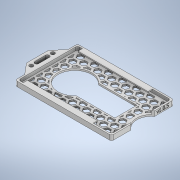
# Autodesk Inventor part: badge
Saved by Autodesk Inventor 2022 (Build 260153000, 153)
## iProperties
Created: 2019-12-22
Part Number: badge
Material: Generic
Document SubType Name: Modeling
Designer: user
Density: 1 g/cm^3
Appearance: Default
Author: user
## iProperties of the stored document _3DPrint.ipt
Created: 2019-12-23
Part Number: _3DPrint
Material: Generic
Document SubType Name: Modeling
Designer: user
Density: 1 g/cm^3
Appearance: Default
Author: user
Autodesk Inventor part; units mm, degrees
(part 1 of 2)
ref_plane "YZ Plane" through (0, 0, 0) normal (1, 0, 0) x (0, 1, 0)
ref_plane "XZ Plane" through (0, 0, 0) normal (0, 1, 0) x (-1, 0, 0)
ref_plane "XY Plane" through (0, 0, 0) normal (0, 0, 1) x (1, 0, 0)
sketch "Sketch1" plane through (0, 0, 0) normal (0, 1, 0) x (-1, 0, 0)
  line L0 (10.6639, 24.1888) -> (-74.7361, 24.1888)
  line L1 (-74.7361, -33.7112) -> (10.6639, -33.7112)
  line L2 (12.6639, 15.2886) -> (20.5717, 5.8644)
  line L3 (21.0396, 4.5789) -> (21.0396, -14.1414)
  line L4 (20.5717, -15.427) -> (12.6639, -24.8511)
  circle A0 centre (-13.8361, -4.7612) radius 17
  line L5 (-62.6217, 4.9888) -> (-62.6217, -14.5112)
  line L6 (-60.6217, -16.5112) -> (-26.1217, -16.5112)
  line L7 (-26.1217, 6.9888) -> (-60.6217, 6.9888)
  arc A1 (-62.6217, -14.5112) -> (-60.6217, -16.5112) centre (-60.6217, -14.5112) ccw
  arc A2 (-60.6217, 6.9888) -> (-62.6217, 4.9888) centre (-60.6217, 4.9888) ccw
  line L8 (-28.5861, -0.5112) -> (-55.1217, -0.5112)
  line L9 (-55.1217, -0.5112) -> (-55.1217, -9.0112)
  line L10 (-55.1217, -9.0112) -> (-28.5861, -9.0112)
  line L11 (-28.5861, -9.0112) -> (-28.5861, -0.5112)
  line L12 (-76.7361, 6.1888) -> (-76.7361, 22.1888)
  line L13 (-76.7361, -15.7112) -> (-76.7361, -31.7112)
  line L14 (9.1639, 22.6888) -> (-73.2361, 22.6888)
  line L15 (-73.2361, -32.2112) -> (9.1639, -32.2112)
  line L16 (11.1639, -30.2112) -> (11.1639, 20.6888)
  line L17 (-75.2361, 20.6888) -> (-75.2361, 4.8633)
  line L18 (-75.2361, -30.2112) -> (-75.2361, -14.3857)
  line L19 (12.6639, 22.1888) -> (12.6639, 15.2886)
  line L20 (12.6639, -24.8511) -> (12.6639, -31.7112)
  arc A3 (-76.7361, -31.7112) -> (-74.7361, -33.7112) centre (-74.7361, -31.7112) ccw
  arc A4 (-75.2361, -30.2112) -> (-73.2361, -32.2112) centre (-73.2361, -30.2112) ccw
  arc A5 (-73.2361, 22.6888) -> (-75.2361, 20.6888) centre (-73.2361, 20.6888) ccw
  arc A6 (-74.7361, 24.1888) -> (-76.7361, 22.1888) centre (-74.7361, 22.1888) ccw
  arc A7 (12.6639, 22.1888) -> (10.6639, 24.1888) centre (10.6639, 22.1888) ccw
  arc A8 (11.1639, 20.6888) -> (9.1639, 22.6888) centre (9.1639, 20.6888) ccw
  arc A9 (9.1639, -32.2112) -> (11.1639, -30.2112) centre (9.1639, -30.2112) ccw
  arc A10 (10.6639, -33.7112) -> (12.6639, -31.7112) centre (10.6639, -31.7112) ccw
  arc A11 (20.5717, -15.427) -> (21.0396, -14.1414) centre (19.0396, -14.1414) ccw
  arc A12 (21.0396, 4.5789) -> (20.5717, 5.8644) centre (19.0396, 4.5789) ccw
  arc A13 (-76.7361, -15.7112) -> (-76.7361, 6.1888) centre (-85.0764, -4.7612) ccw
  circle A14 centre (16.6641, 5.1661) radius 1.75
  circle A15 centre (16.6641, -14.7286) radius 1.75
  line L21 (12.6639, 15.2886) -> (12.6639, -24.8511)
  line L22 (18.4257, 0.4632) -> (18.4257, -9.9334)
  line L23 (14.9257, 0.4403) -> (14.9257, -10.0946)
  arc A16 (14.9257, -10.0946) -> (18.4257, -9.9334) centre (16.6641, -9.7623) ccw
  arc A17 (18.4257, 0.4632) -> (14.9257, 0.4403) centre (16.6774, 0.1997) ccw
  point P0 (0, 0)
  point P1 (12.6639, 24.1888)
  point P2 (-76.7361, -33.7112)
  point P3 (-76.7361, 24.1888)
  point P4 (12.6639, -33.7112)
  point P5 (21.0396, -14.8693)
  point P6 (-62.6217, -16.5112)
  dimension "d19" = 18
  dimension "d20" = 34
  dimension "d26" = 2
  dimension "d28" = 7.5
  dimension "d32" = 7.5
  dimension "d33" = 7.5
  dimension "d36" = 1.5
  dimension "d37" = 1.5
  dimension "d40" = 1.5
  dimension "d41" = 2
  dimension "d84" = 54.9
  dimension "d89" = 18
  dimension "d104" = 86.4
  dimension "d110" = 13.7646
  dimension "d116" = 1.5
  dimension "d122" = 3.5
  dimension "d123" = 3.5
  dimension "d124" = 3.4423
  dimension "d125" = 3.4423
  dimension "d155" = 25
  dimension "d163" = 15.7
  dimension "d164" = 15.7
  dimension "d165" = 27.45
  dimension "d166" = 27.45
  dimension "d167" = 8.5
  dimension "d171" = 26.5357
  dimension "d173" = 39.75
  dimension "d213" = 4.0002
  dimension "d214" = 4.0002
  dimension "d219" = 140
  dimension "d221" = 140
  dimension "d246" = 4.9664
  dimension "d247" = 4.9664
  dimension "d248" = 13.5
  dimension "d249" = 1.5
  dimension "d250" = 1.5
  dimension "d251" = 4.0002
  dimension "d262" = 3.5
  dimension "d263" = 2.6139
  constraints: 48 end point, 34 point on circle, 24 tangent, 18 centre point, 13 point on line, 10 equal radius, 6 vertical, 5 parallel, 3 horizontal, 3 perpendicular, 2 collinear
  measures "d19" distance of point (-76.736, 24.189) L12.start
  measures "d20" diameter of A0
  measures "d26" radius of A1
  measures "d28" distance between parallel lines of L6 L10
  measures "d32" distance between parallel lines of L8 L7
  measures "d33" distance between parallel lines of L5 L9
  measures "d36" distance between parallel lines of L0 L14
  measures "d37" distance between parallel lines of L1 L15
  measures "d40" distance between parallel lines of L13 L18
  measures "d41" radius of A3
  measures "d84" distance between parallel lines of L15 L14
  measures "d89" distance of L13.start point (-76.736, -33.711)
  measures "d104" distance between parallel lines of L17 L16
  measures "d110" radius of A13
  measures "d116" distance between parallel lines of L17 L12
  measures "d122" diameter of A15
  measures "d123" diameter of A14
  measures "d124" distance from line of L4 A15.centre
  measures "d125" distance from line of L2 A14.centre
  measures "d155" distance from line of L16 A0.centre
  measures "d163" distance between parallel lines of L15 L6
  measures "d164" distance between parallel lines of L14 L7
  measures "d165" distance from line of L15 A0.centre
  measures "d166" distance from line of L14 A0.centre
  measures "d167" distance between parallel lines of L8 L10
  measures "d171" distance between parallel lines of L9 L11
  measures "d173" distance between parallel lines of L16 L11
  measures "d213" distance from line of L21 A14.centre
  measures "d214" distance from line of L21 A15.centre
  measures "d219" angle of L19 L2
  measures "d221" angle of L20 L4
  measures "d246" distance of A17.centre A14.centre
  measures "d247" distance of A15.centre A16.centre
  measures "d249" distance between parallel lines of L16 L19
  measures "d250" distance between parallel lines of L16 L20
  measures "d251" distance from line of L21 A16.centre
  measures "d262" distance between parallel lines of L23 L22
  measures "d263" distance from line of L3 L22.end
extrude "OutsideFrame_Ex" add sketch "Sketch1" along normal blind 4.5 contours A7 L19 L21 L20 A10 L1 A3 L13 A13 L18 A4 L15 A9 L16 A8 L14 A5 L17 L12 A6 L0
extrude "CardRidge" add sketch "Sketch1" along normal blind 1.5 contours L17 A5 L14 A8 L16 A9 L15 A4 L18 A13 | A0 L10 L11 L8 | A0 L8 L9 L10 L6 A1 L5 A2 L7 picked at (-18.0028, -4.7612)
sketch "Sketch5" plane through (73.2361, 4.5, 22.6888) normal (0, 0, -1) x (-1, 0, 0)
  line L0 (-2, 0) -> (0, 0) projected
  line L1 (79.9, 0) -> (79.9, -1)
  line L2 (0, 0) -> (82.4, 0) projected
  line L3 (15, 0) -> (79.9, 0)
  line L4 (79.9, 0) -> (79.9, -1)
  line L5 (79.9, -1) -> (15, -1)
  line L6 (15, -1) -> (15, 0)
  line L7 (0, -4.5) -> (0, 0) projected
  line L8 (82.4, -4.5) -> (82.4, 0) projected
  line L9 (0, -3) -> (82.4, -3) projected
  point P0 (73.2361, -4.5)
  dimension "d65" = 15
  dimension "d66" = 2.5
  dimension "d67" = 1
  constraints: 10 end point, 2 parallel, 1 horizontal, 1 perpendicular, 1 point on line
  measures "d65" distance between parallel lines of L7 L6
  measures "d66" distance between parallel lines of L8 L1
  measures "d67" distance between parallel lines of L5 L2
extrude "LeftSlider" add sketch "Sketch5" along normal blind 4 contours L1 L5 L6 L2
sketch "Sketch6" plane through (-9.1639, 4.5, -32.2112) normal (0, 0, 1) x (1, 0, 0)
  line L0 (83.9, 0) -> (-1.5, 0) projected
  line L1 (2.5, 0) -> (67.4, 0)
  line L2 (67.4, 0) -> (67.4, -1)
  line L3 (67.4, -1) -> (2.5, -1)
  line L4 (2.5, -1) -> (2.5, 0)
  line L5 (0, -3) -> (0, 0) projected
  line L6 (82.4, -3) -> (82.4, 0) projected
  point P0 (9.1639, -4.5)
  point P1 (0, -7.4)
  point P2 (83.7968, -7.4)
  dimension "d71" = 2.5
  dimension "d72" = 15
  dimension "d73" = 1
  constraints: 8 end point, 2 parallel, 1 horizontal, 1 perpendicular, 1 point on line, 1 other
  measures "d71" distance between parallel lines of L5 L4
  measures "d73" distance between parallel lines of L3 L0
extrude "RightSlider" add sketch "Sketch6" along normal blind 4
extrude "TopHolder" add sketch "Sketch1" along normal blind 4.5 contours L2 A12 L3 A11 L4 L21
sketch "Sketch15" plane through (76.7361, 0, -15.7112) normal (1, 0, 0) x (0, 0, -1)
  line L0 (2.0176, 4.0473) -> (13.0095, 4.0473) construction
  line L1 (13.0095, 4.0473) -> (13.0095, -1.0349) construction
  line L2 (13.0095, -1.0349) -> (2.0176, -1.0349) construction
  line L3 (2.0176, -1.0349) -> (2.0176, 4.0473) construction
  line L4 (4.0924, 3.2248) -> (3.2304, 0.9376)
  line L5 (3.2304, 0.9376) -> (2.8846, 0.9376)
  line L6 (2.8846, 0.9376) -> (2.03, 3.2248)
  line L7 (2.03, 3.2248) -> (2.4474, 3.2248)
  line L8 (2.4474, 3.2248) -> (3.0723, 1.4637)
  line L9 (3.0723, 1.4637) -> (3.6923, 3.2248)
  line L10 (3.6923, 3.2248) -> (4.0924, 3.2248)
  line L11 (6.0536, 0.9376) -> (4.5667, 0.9376)
  line L12 (4.5667, 0.9376) -> (4.5667, 1.2488)
  line L13 (4.5667, 1.2488) -> (5.1199, 1.2488)
  line L14 (5.1199, 1.2488) -> (5.1199, 3.2915)
  line L15 (5.1199, 3.2915) -> (4.5667, 3.2915)
  line L16 (4.5667, 3.2915) -> (4.5667, 3.5706)
  spline S0 degree 2 poles (4.5667, 3.5706) (4.8803, 3.5706) (5.1768, 3.7485) (5.1965, 3.9955) knots 0 0 0 1 2 2 2
  line L17 (5.1965, 3.9955) -> (5.5127, 3.9955)
  line L18 (5.5127, 3.9955) -> (5.5127, 1.2488)
  line L19 (5.5127, 1.2488) -> (6.0536, 1.2488)
  line L20 (6.0536, 1.2488) -> (6.0536, 0.9376)
  line L21 (7.2689, 0.9376) -> (6.7798, 0.9376)
  line L22 (6.7798, 0.9376) -> (6.7798, 1.5205)
  line L23 (6.7798, 1.5205) -> (7.2689, 1.5205)
  line L24 (7.2689, 1.5205) -> (7.2689, 0.9376)
  spline S1 degree 2 poles (9.7809, 2.4616) (9.7809, 1.6415) (9.3041, 0.8734) (8.8077, 0.8734) knots 0 0 0 1 2 2 2
  spline S2 degree 2 poles (8.8077, 0.8734) (8.3038, 0.8734) (7.832, 1.6564) (7.832, 2.4591) knots 0 0 0 1 2 2 2
  spline S3 degree 2 poles (7.832, 2.4591) (7.832, 3.2841) (8.3087, 4.0473) (8.8077, 4.0473) knots 0 0 0 1 2 2 2
  spline S4 degree 2 poles (8.8077, 4.0473) (9.3091, 4.0473) (9.7809, 3.2569) (9.7809, 2.4616) knots 0 0 0 1 2 2 2
  spline S5 degree 2 poles (9.2572, 1.5329) (9.3165, 1.6835) (9.3659, 2.1479) (9.3659, 2.4616) knots 0 0 0 1 2 2 2
  spline S6 degree 2 poles (9.3659, 2.4616) (9.3659, 2.7753) (9.3165, 3.2372) (9.2547, 3.3928) knots 0 0 0 1 2 2 2
  spline S7 degree 2 poles (9.2547, 3.3928) (9.193, 3.5484) (8.9781, 3.7089) (8.8077, 3.7089) knots 0 0 0 1 2 2 2
  spline S8 degree 2 poles (8.8077, 3.7089) (8.6372, 3.7089) (8.4174, 3.5484) (8.3532, 3.3878) knots 0 0 0 1 2 2 2
  spline S9 degree 2 poles (8.3532, 3.3878) (8.2914, 3.2322) (8.247, 2.758) (8.247, 2.4591) knots 0 0 0 1 2 2 2
  spline S10 degree 2 poles (8.247, 2.4591) (8.247, 2.138) (8.2865, 1.7082) (8.3507, 1.5403) knots 0 0 0 1 2 2 2
  spline S11 degree 2 poles (8.3507, 1.5403) (8.41, 1.3822) (8.6298, 1.2118) (8.8077, 1.2118) knots 0 0 0 1 2 2 2
  spline S12 degree 2 poles (8.8077, 1.2118) (8.9756, 1.2118) (9.1955, 1.3723) (9.2572, 1.5329) knots 0 0 0 1 2 2 2
  line L25 (10.8257, 0.9376) -> (10.3366, 0.9376)
  line L26 (10.3366, 0.9376) -> (10.3366, 1.5205)
  line L27 (10.3366, 1.5205) -> (10.8257, 1.5205)
  line L28 (10.8257, 1.5205) -> (10.8257, 0.9376)
  spline S13 degree 2 poles (13.2883, 1.9058) (13.2883, 1.686) (13.1475, 1.3106) (13.0191, 1.1722) knots 0 0 0 1 2 2 2
  spline S14 degree 2 poles (13.0191, 1.1722) (12.8906, 1.0339) (12.5078, 0.8734) (12.2706, 0.8734) knots 0 0 0 1 2 2 2
  spline S15 degree 2 poles (12.2706, 0.8734) (12.0533, 0.8734) (11.6284, 0.9697) (11.4728, 1.0463) knots 0 0 0 1 2 2 2
  line L29 (11.4728, 1.0463) -> (11.4728, 1.4785)
  line L30 (11.4728, 1.4785) -> (11.5025, 1.4785)
  spline S16 degree 2 poles (11.5025, 1.4785) (11.5494, 1.4439) (11.7248, 1.355) (11.831, 1.3155) knots 0 0 0 1 2 2 2
  spline S17 degree 2 poles (11.831, 1.3155) (11.952, 1.2735) (12.1521, 1.2266) (12.278, 1.2266) knots 0 0 0 1 2 2 2
  spline S18 degree 2 poles (12.278, 1.2266) (12.4015, 1.2266) (12.6337, 1.3155) (12.7177, 1.4118) knots 0 0 0 1 2 2 2
  spline S19 degree 2 poles (12.7177, 1.4118) (12.7943, 1.5032) (12.8733, 1.7453) (12.8733, 1.9083) knots 0 0 0 1 2 2 2
  spline S20 degree 2 poles (12.8733, 1.9083) (12.8733, 2.0713) (12.7844, 2.2788) (12.7004, 2.348) knots 0 0 0 1 2 2 2
  spline S21 degree 2 poles (12.7004, 2.348) (12.614, 2.4245) (12.3571, 2.4888) (12.2015, 2.4888) knots 0 0 0 1 2 2 2
  spline S22 degree 2 poles (12.2015, 2.4888) (12.0335, 2.4888) (11.7001, 2.4369) (11.5988, 2.4147) knots 0 0 0 1 2 2 2
  line L31 (11.5988, 2.4147) -> (11.5988, 3.9856)
  line L32 (11.5988, 3.9856) -> (13.271, 3.9856)
  line L33 (13.271, 3.9856) -> (13.271, 3.6274)
  line L34 (13.271, 3.6274) -> (11.9915, 3.6274)
  line L35 (11.9915, 3.6274) -> (11.9915, 2.8148)
  spline S23 degree 2 poles (11.9915, 2.8148) (12.0656, 2.8247) (12.2089, 2.8321) (12.2682, 2.8321) knots 0 0 0 1 2 2 2
  spline S24 degree 2 poles (12.2682, 2.8321) (12.5028, 2.8321) (12.8264, 2.7555) (12.9746, 2.6419) knots 0 0 0 1 2 2 2
  spline S25 degree 2 poles (12.9746, 2.6419) (13.1253, 2.5283) (13.2883, 2.1825) (13.2883, 1.9058) knots 0 0 0 1 2 2 2
  point P0 (-15.7112, 0)
  constraints: 2 other
emboss "VersionNumber" sketch "Sketch15" operation cut depth 1 direction (-1, 0, 0)
sketch "Sketch21" plane through (0, 1.5, 0) normal (0, 1, 0) x (1, 0, 0)
  line L0 (-1.084, -12.9121) -> (-5.3551, -12.9839)
  line L1 (-5.3551, -12.9839) -> (-7.5528, -9.321)
  line L2 (-7.5528, -9.321) -> (-5.4795, -5.5862)
  line L3 (-5.4795, -5.5862) -> (-1.2085, -5.5144)
  line L4 (-1.2085, -5.5144) -> (0.9893, -9.1773)
  line L5 (0.9893, -9.1773) -> (-1.084, -12.9121)
  line L6 (-1.3329, 1.8833) -> (-5.604, 1.8114)
  line L7 (-5.604, 1.8114) -> (-7.6773, -1.9233)
  line L8 (-7.6773, -1.9233) -> (-5.4795, -5.5862)
  line L9 (-1.2085, -5.5144) -> (0.8649, -1.7796)
  line L10 (0.8649, -1.7796) -> (-1.3329, 1.8833)
  line L11 (-1.6781, -11.9219) -> (-4.7946, -11.9744)
  line L12 (-4.7946, -11.9744) -> (-6.3983, -9.3016)
  line L13 (-6.3983, -9.3016) -> (-4.8854, -6.5764)
  line L14 (-4.8854, -6.5764) -> (-1.7689, -6.524)
  line L15 (-1.7689, -6.524) -> (-0.1652, -9.1967)
  line L16 (-0.1652, -9.1967) -> (-1.6781, -11.9219)
  line L17 (-1.8025, -4.5242) -> (-4.9191, -4.5767)
  line L18 (-4.9191, -4.5767) -> (-6.5227, -1.9039)
  line L19 (-6.5227, -1.9039) -> (-5.0099, 0.8213)
  line L20 (-5.0099, 0.8213) -> (-1.8933, 0.8737)
  line L21 (-1.8933, 0.8737) -> (-0.2897, -1.799)
  line L22 (-0.2897, -1.799) -> (-1.8025, -4.5242)
  line L23 (-5.7284, 9.2091) -> (-1.4573, 9.281)
  line L24 (-5.604, 1.8114) -> (-7.8017, 5.4744)
  line L25 (-7.8017, 5.4744) -> (-5.7284, 9.2091)
  line L26 (-1.4573, 9.281) -> (0.7404, 5.6181)
  line L27 (0.7404, 5.6181) -> (-1.3329, 1.8833)
  line L28 (-2.0178, 8.2714) -> (-5.1343, 8.219)
  line L29 (-5.1343, 8.219) -> (-6.6472, 5.4938)
  line L30 (-6.6472, 5.4938) -> (-5.0435, 2.821)
  line L31 (-5.0435, 2.821) -> (-1.927, 2.8734)
  line L32 (-1.927, 2.8734) -> (-0.4141, 5.5986)
  line L33 (-0.4141, 5.5986) -> (-2.0178, 8.2714)
  line L34 (-1.5818, 16.6787) -> (-5.8528, 16.6068)
  line L35 (-2.0514, 10.2711) -> (-5.1679, 10.2187)
  line L36 (-5.1679, 10.2187) -> (-6.7716, 12.8915)
  line L37 (-0.5386, 12.9963) -> (-2.0514, 10.2711)
  line L38 (-7.9261, 12.872) -> (-5.7284, 9.2091)
  line L39 (-1.4573, 9.281) -> (0.616, 13.0157)
  line L40 (-5.2588, 15.6167) -> (-2.1422, 15.6691)
  line L41 (-2.1422, 15.6691) -> (-0.5386, 12.9963)
  line L42 (0.616, 13.0157) -> (-1.5818, 16.6787)
  line L43 (-6.7716, 12.8915) -> (-5.2588, 15.6167)
  line L44 (-5.8528, 16.6068) -> (-7.9261, 12.872)
  line L45 (5.1359, -1.7078) -> (7.3337, -5.3707)
  line L46 (7.3337, -5.3707) -> (11.6047, -5.2988)
  line L47 (-1.3329, 1.8833) -> (0.7404, 5.6181)
  line L48 (5.1359, -1.7078) -> (0.8649, -1.7796)
  line L49 (-5.7284, 9.2091) -> (-7.8017, 5.4744)
  line L50 (-6.6472, 5.4938) -> (-5.1343, 8.219)
  line L51 (-5.1343, 8.219) -> (-2.0178, 8.2714)
  line L52 (-5.0435, 2.821) -> (-6.6472, 5.4938)
  line L53 (-1.4573, 9.281) -> (-5.7284, 9.2091)
  line L54 (-7.8017, 5.4744) -> (-5.604, 1.8114)
  line L55 (-0.4141, 5.5986) -> (-1.927, 2.8734)
  line L56 (-1.927, 2.8734) -> (-5.0435, 2.821)
  line L57 (-5.604, 1.8114) -> (-1.3329, 1.8833)
  line L58 (-2.0178, 8.2714) -> (-0.4141, 5.5986)
  line L59 (0.7404, 5.6181) -> (-1.4573, 9.281)
  line L60 (-11.6031, 11.81) -> (-13.116, 9.0848)
  line L61 (-8.4866, 11.8625) -> (-11.6031, 11.81)
  line L62 (-13.116, 9.0848) -> (-11.5123, 6.4121)
  line L63 (-12.1972, 12.8002) -> (-7.9261, 12.872)
  line L64 (-8.3958, 6.4645) -> (-6.8829, 9.1897)
  line L65 (-11.5123, 6.4121) -> (-8.3958, 6.4645)
  line L66 (-7.8017, 5.4744) -> (-12.0728, 5.4025)
  line L67 (-6.8829, 9.1897) -> (-8.4866, 11.8625)
  line L68 (-12.0728, 5.4025) -> (-14.2705, 9.0654)
  line L69 (-14.2705, 9.0654) -> (-12.1972, 12.8002)
  line L70 (32.7111, 9.8558) -> (30.5133, 13.5187)
  line L71 (30.5133, 13.5187) -> (26.2423, 13.4468)
  line L72 (17.7008, 13.2313) -> (19.7735, 17.0379)
  line L73 (19.7735, 17.0379) -> (24.0445, 17.1097)
  line L74 (24.0445, 17.1097) -> (26.2423, 13.4468)
  line L75 (13.3047, 20.629) -> (11.2314, 16.8942)
  line L76 (12.3859, 16.9136) -> (13.8988, 19.6388)
  line L77 (13.8988, 19.6388) -> (17.0153, 19.6912)
  line L78 (13.9896, 14.2409) -> (12.3859, 16.9136)
  line L79 (17.5757, 20.7008) -> (13.3047, 20.629)
  line L80 (11.2314, 16.8942) -> (13.4291, 13.2313)
  line L81 (18.6189, 17.0185) -> (17.1061, 14.2933)
  line L82 (17.1061, 14.2933) -> (13.9896, 14.2409)
  line L83 (17.0153, 19.6912) -> (18.6189, 17.0185)
  line L84 (19.7735, 17.0379) -> (17.5757, 20.7008)
  line L85 (7.43, 23.2299) -> (5.9171, 20.5047)
  line L86 (10.5465, 23.2823) -> (7.43, 23.2299)
  line L87 (5.9171, 20.5047) -> (7.5208, 17.8319)
  line L88 (6.8359, 24.22) -> (11.1069, 24.2919)
  line L89 (10.6373, 17.8844) -> (12.1501, 20.6095)
  line L90 (7.5208, 17.8319) -> (10.6373, 17.8844)
  line L91 (11.2314, 16.8942) -> (6.9603, 16.8224)
  line L92 (12.1501, 20.6095) -> (10.5465, 23.2823)
  line L93 (11.1069, 24.2919) -> (13.3047, 20.629)
  line L94 (6.9603, 16.8224) -> (4.7626, 20.4853)
  line L95 (4.7626, 20.4853) -> (6.8359, 24.22)
  line L96 (13.9896, 14.2409) -> (17.1061, 14.2933)
  line L97 (12.3859, 16.9136) -> (13.9896, 14.2409)
  line L98 (17.1061, 14.2933) -> (18.6189, 17.0185)
  line L99 (13.4291, 13.2313) -> (11.2314, 16.8942)
  line L100 (19.7735, 17.0379) -> (17.7008, 13.2313)
  line L101 (17.0153, 19.6912) -> (13.8988, 19.6388)
  line L102 (13.8988, 19.6388) -> (12.3859, 16.9136)
  line L103 (11.2314, 16.8942) -> (13.3047, 20.629)
  line L104 (13.3047, 20.629) -> (17.5757, 20.7008)
  line L105 (18.6189, 17.0185) -> (17.0153, 19.6912)
  line L106 (17.5757, 20.7008) -> (19.7735, 17.0379)
  line L107 (0.7404, 5.6181) -> (-1.4573, 9.281)
  line L108 (6.9603, 16.8224) -> (11.2314, 16.8942)
  line L109 (11.2314, 16.8942) -> (13.4291, 13.2313)
  line L110 (-5.3551, -12.9839) -> (-7.4284, -16.7187)
  line L111 (-7.4284, -16.7187) -> (-5.2306, -20.3816)
  line L112 (-5.2306, -20.3816) -> (-0.9596, -20.3098)
  line L113 (-0.9596, -20.3098) -> (1.1137, -16.575)
  line L114 (1.1137, -16.575) -> (-1.084, -12.9121)
  line L115 (-1.6445, -13.9216) -> (-4.761, -13.9741)
  line L116 (-4.761, -13.9741) -> (-6.2738, -16.6993)
  line L117 (-6.2738, -16.6993) -> (-4.6702, -19.372)
  line L118 (-4.6702, -19.372) -> (-1.5536, -19.3196)
  line L119 (-1.5536, -19.3196) -> (-0.0408, -16.5944)
  line L120 (-0.0408, -16.5944) -> (-1.6445, -13.9216)
  line L121 (-7.5528, -9.321) -> (-5.3551, -12.9839)
  line L122 (-11.8239, -9.3929) -> (-7.5528, -9.321)
  line L123 (-11.2298, -10.383) -> (-8.1133, -10.3306)
  line L124 (-12.7426, -13.1082) -> (-11.2298, -10.383)
  line L125 (-13.8972, -13.1276) -> (-11.8239, -9.3929)
  line L126 (-11.139, -15.781) -> (-12.7426, -13.1082)
  line L127 (-11.6994, -16.7905) -> (-13.8972, -13.1276)
  line L128 (-7.4284, -16.7187) -> (-11.6994, -16.7905)
  line L129 (-8.0225, -15.7285) -> (-11.139, -15.781)
  line L130 (-6.5096, -13.0033) -> (-8.0225, -15.7285)
  line L131 (-8.1133, -10.3306) -> (-6.5096, -13.0033)
  line L132 (-0.8351, -27.7074) -> (-5.1062, -27.7793)
  line L133 (1.2382, -23.9727) -> (-0.8351, -27.7074)
  line L134 (0.0837, -23.9921) -> (-1.4292, -26.7173)
  line L135 (-1.52, -21.3193) -> (0.0837, -23.9921)
  line L136 (-0.9596, -20.3098) -> (1.2382, -23.9727)
  line L137 (-4.6365, -21.3718) -> (-1.52, -21.3193)
  line L138 (-7.3039, -24.1164) -> (-5.2306, -20.3816)
  line L139 (-6.1494, -24.0969) -> (-4.6365, -21.3718)
  line L140 (-4.5457, -26.7697) -> (-6.1494, -24.0969)
  line L141 (-5.1062, -27.7793) -> (-7.3039, -24.1164)
  line L142 (-1.4292, -26.7173) -> (-4.5457, -26.7697)
  line L143 (-13.7727, -20.5253) -> (-11.6994, -16.7905)
  line L144 (-11.575, -24.1882) -> (-13.7727, -20.5253)
  line L145 (-11.0145, -23.1786) -> (-12.6182, -20.5059)
  line L146 (-7.3039, -24.1164) -> (-11.575, -24.1882)
  line L147 (-6.3851, -20.401) -> (-7.898, -23.1262)
  line L148 (-5.2306, -20.3816) -> (-7.3039, -24.1164)
  line L149 (-7.9888, -17.7283) -> (-6.3851, -20.401)
  line L150 (-11.1053, -17.7807) -> (-7.9888, -17.7283)
  line L151 (-11.6994, -16.7905) -> (-7.4284, -16.7187)
  line L152 (-12.6182, -20.5059) -> (-11.1053, -17.7807)
  line L153 (-11.9483, -1.9952) -> (-14.1461, 1.6677)
  line L154 (-7.8017, 5.4744) -> (-5.604, 1.8114)
  line L155 (-7.6773, -1.9233) -> (-11.9483, -1.9952)
  line L156 (-14.1461, 1.6677) -> (-12.0728, 5.4025)
  line L157 (-12.0728, 5.4025) -> (-7.8017, 5.4744)
  line L158 (-12.9915, 1.6872) -> (-11.3879, -0.9856)
  line L159 (-11.3879, -0.9856) -> (-8.2713, -0.9332)
  line L160 (-8.2713, -0.9332) -> (-6.7585, 1.792)
  line L161 (-6.7585, 1.792) -> (-8.3621, 4.4648)
  line L162 (-8.3621, 4.4648) -> (-11.4787, 4.4124)
  line L163 (-11.4787, 4.4124) -> (-12.9915, 1.6872)
  line L164 (-14.0216, -5.7299) -> (-11.8239, -9.3929)
  line L165 (-11.8239, -9.3929) -> (-7.5528, -9.321)
  line L166 (-5.4795, -5.5862) -> (-7.6773, -1.9233)
  line L167 (-7.6773, -1.9233) -> (-11.9483, -1.9952)
  line L168 (-11.9483, -1.9952) -> (-14.0216, -5.7299)
  line L169 (-12.8671, -5.7105) -> (-11.2634, -8.3833)
  line L170 (-11.2634, -8.3833) -> (-8.1469, -8.3309)
  line L171 (-8.1469, -8.3309) -> (-6.634, -5.6057)
  line L172 (-6.634, -5.6057) -> (-8.2377, -2.9329)
  line L173 (-8.2377, -2.9329) -> (-11.3542, -2.9853)
  line L174 (-11.3542, -2.9853) -> (-12.8671, -5.7105)
  line L175 (-0.2897, -1.799) -> (-1.8933, 0.8737)
  line L176 (0.8649, -1.7796) -> (5.1359, -1.7078)
  line L177 (5.2604, -9.1055) -> (0.9893, -9.1773)
  line L178 (0.9893, -9.1773) -> (-1.2085, -5.5144)
  line L179 (-1.2085, -5.5144) -> (0.8649, -1.7796)
  line L180 (7.3337, -5.3707) -> (5.2604, -9.1055)
  line L181 (1.4589, -2.7698) -> (4.5755, -2.7173)
  line L182 (-0.0539, -5.495) -> (1.4589, -2.7698)
  line L183 (6.1791, -5.3901) -> (4.6663, -8.1153)
  line L184 (4.6663, -8.1153) -> (1.5497, -8.1677)
  line L185 (1.5497, -8.1677) -> (-0.0539, -5.495)
  line L186 (4.5755, -2.7173) -> (6.1791, -5.3901)
  line L187 (51.7442, 21.2756) -> (49.5464, 24.9385)
  line L188 (36.9821, 9.9276) -> (32.7111, 9.8558)
  line L189 (33.1471, 18.263) -> (31.5434, 20.9358)
  line L190 (30.3889, 20.9164) -> (32.5866, 17.2534)
  line L191 (36.2636, 18.3154) -> (33.1471, 18.263)
  line L192 (32.5866, 17.2534) -> (36.8577, 17.3253)
  line L193 (33.1807, 16.2633) -> (36.2972, 16.3157)
  line L194 (30.5133, 13.5187) -> (32.5866, 17.2534)
  line L195 (31.6679, 13.5381) -> (33.1807, 16.2633)
  line L196 (33.2715, 10.8653) -> (31.6679, 13.5381)
  line L197 (36.388, 10.9178) -> (33.2715, 10.8653)
  line L198 (36.8577, 17.3253) -> (39.0554, 13.6624)
  line L199 (39.0554, 13.6624) -> (36.9821, 9.9276)
  line L200 (37.8878, 24.7424) -> (39.4914, 22.0696)
  line L201 (38.931, 21.0601) -> (36.7964, 24.6886)
  line L202 (36.1728, 23.7134) -> (37.7765, 21.0406)
  line L203 (37.7765, 21.0406) -> (36.2636, 18.3154)
  line L204 (36.8577, 17.3253) -> (38.931, 21.0601)
  line L205 (36.2972, 16.3157) -> (37.9009, 13.643)
  line L206 (37.9009, 13.643) -> (36.388, 10.9178)
  line L207 (31.5434, 20.9358) -> (33.0563, 23.661)
  line L208 (32.4622, 24.6511) -> (30.3889, 20.9164)
  line L209 (33.0226, 25.6607) -> (31.419, 28.3335)
  line L210 (30.2644, 28.314) -> (32.4622, 24.6511)
  line L211 (32.4622, 24.6511) -> (30.2644, 28.314)
  line L212 (31.419, 28.3335) -> (33.0226, 25.6607)
  line L213 (32.9318, 31.0587) -> (31.419, 28.3335)
  line L214 (30.2644, 28.314) -> (32.3377, 32.0488)
  line L215 (32.3377, 32.0488) -> (36.6088, 32.1207)
  line L216 (39.4006, 27.4676) -> (37.8878, 24.7424)
  line L217 (39.4914, 22.0696) -> (42.608, 22.1221)
  line L218 (43.202, 21.1319) -> (38.931, 21.0601)
  line L219 (42.608, 22.1221) -> (44.1208, 24.8473)
  line L220 (45.2754, 24.8667) -> (43.202, 21.1319)
  line L221 (42.5172, 27.52) -> (39.4006, 27.4676)
  line L222 (44.1208, 24.8473) -> (42.5172, 27.52)
  line L223 (43.0776, 28.5296) -> (45.2754, 24.8667)
  line L224 (38.8065, 28.4577) -> (43.0776, 28.5296)
  line L225 (49.6709, 17.5408) -> (51.7442, 21.2756)
  line L226 (45.8694, 23.8765) -> (44.3566, 21.1513)
  line L227 (48.986, 23.929) -> (45.8694, 23.8765)
  line L228 (43.202, 21.1319) -> (45.3998, 17.469)
  line L229 (44.3566, 21.1513) -> (45.9602, 18.4786)
  line L230 (50.5896, 21.2562) -> (48.986, 23.929)
  line L231 (45.9602, 18.4786) -> (49.0768, 18.531)
  line L232 (49.0768, 18.531) -> (50.5896, 21.2562)
  line L233 (45.3998, 17.469) -> (49.6709, 17.5408)
  line L234 (36.7964, 24.6886) -> (32.4622, 24.6511)
  line L235 (33.0563, 23.661) -> (36.1728, 23.7134)
  line L236 (33.0226, 25.6607) -> (36.1392, 25.7131)
  line L237 (36.1392, 25.7131) -> (33.0226, 25.6607)
  line L238 (32.4622, 24.6511) -> (36.7964, 24.6886)
  line L239 (36.1392, 25.7131) -> (37.652, 28.4383)
  line L240 (36.7964, 24.6886) -> (38.8065, 28.4577)
  line L241 (36.0484, 31.1111) -> (32.9318, 31.0587)
  line L242 (36.0484, 31.1111) -> (37.652, 28.4383)
  line L243 (49.5464, 24.9385) -> (45.2754, 24.8667)
  line L244 (36.6088, 32.1207) -> (38.8065, 28.4577)
  line L245 (38.0122, 17.3447) -> (39.6159, 14.672)
  line L246 (38.931, 21.0601) -> (36.8577, 17.3253)
  line L247 (43.202, 21.1319) -> (38.931, 21.0601)
  line L248 (42.6416, 20.1223) -> (39.5251, 20.0699)
  line L249 (45.3998, 17.469) -> (43.202, 21.1319)
  line L250 (44.2453, 17.4496) -> (42.6416, 20.1223)
  line L251 (39.6159, 14.672) -> (42.7324, 14.7244)
  line L252 (39.0554, 13.6624) -> (43.3265, 13.7342)
  line L253 (42.7324, 14.7244) -> (44.2453, 17.4496)
  line L254 (43.3265, 13.7342) -> (45.3998, 17.469)
  line L255 (39.5251, 20.0699) -> (38.0122, 17.3447)
  line L256 (32.5866, 17.2534) -> (30.5133, 13.5187)
  line L257 (45.5242, 10.0713) -> (49.7953, 10.1432)
  line L258 (36.388, 10.9178) -> (37.9009, 13.643)
  line L259 (36.9821, 9.9276) -> (39.0554, 13.6624)
  line L260 (43.3265, 13.7342) -> (45.5242, 10.0713)
  line L261 (36.8577, 17.3253) -> (32.5866, 17.2534)
  line L262 (32.7111, 9.8558) -> (36.9821, 9.9276)
  line L263 (33.2715, 10.8653) -> (36.388, 10.9178)
  line L264 (30.5133, 13.5187) -> (32.7111, 9.8558)
  line L265 (31.6679, 13.5381) -> (33.2715, 10.8653)
  line L266 (33.1807, 16.2633) -> (31.6679, 13.5381)
  line L267 (37.9009, 13.643) -> (36.2972, 16.3157)
  line L268 (39.0554, 13.6624) -> (36.8577, 17.3253)
  line L269 (36.2972, 16.3157) -> (33.1807, 16.2633)
  line L270 (39.3043, -1.133) -> (43.5754, -1.0611)
  line L271 (37.231, -4.8677) -> (39.3043, -1.133)
  line L272 (30.7622, -1.2767) -> (32.96, -4.9396)
  line L273 (32.96, -4.9396) -> (37.231, -4.8677)
  line L274 (30.7622, -1.2767) -> (26.4912, -1.3485)
  line L275 (24.4179, -5.0833) -> (20.1468, -5.1551)
  line L276 (24.4179, -5.0833) -> (26.4912, -1.3485)
  line L277 (24.4179, -5.0833) -> (26.6156, -8.7462)
  line L278 (25.5724, -5.0639) -> (27.0853, -2.3387)
  line L279 (26.4912, -1.3485) -> (24.4179, -5.0833)
  line L280 (30.2018, -2.2863) -> (27.0853, -2.3387)
  line L281 (30.7622, -1.2767) -> (26.4912, -1.3485)
  line L282 (31.8054, -4.959) -> (30.2018, -2.2863)
  line L283 (30.2926, -7.6842) -> (31.8054, -4.959)
  line L284 (32.96, -4.9396) -> (30.8867, -8.6744)
  line L285 (30.2926, -7.6842) -> (27.1761, -7.7366)
  line L286 (30.8867, -8.6744) -> (26.6156, -8.7462)
  line L287 (25.5724, -5.0639) -> (27.1761, -7.7366)
  line L288 (13.8025, -8.9618) -> (11.6047, -5.2988)
  line L289 (18.0735, -8.8899) -> (20.1468, -5.1551)
  line L290 (18.0735, -8.8899) -> (13.8025, -8.9618)
  line L291 (18.0735, -8.8899) -> (20.2713, -12.5528)
  line L292 (24.4179, -5.0833) -> (20.1468, -5.1551)
  line L293 (19.2281, -8.8705) -> (20.7409, -6.1453)
  line L294 (18.0735, -8.8899) -> (20.1468, -5.1551)
  line L295 (23.8574, -6.0929) -> (20.7409, -6.1453)
  line L296 (23.9482, -11.4908) -> (25.4611, -8.7656)
  line L297 (24.5423, -12.481) -> (26.6156, -8.7462)
  line L298 (20.8317, -11.5433) -> (19.2281, -8.8705)
  line L299 (23.9482, -11.4908) -> (20.8317, -11.5433)
  line L300 (20.2713, -12.5528) -> (24.5423, -12.481)
  line L301 (23.8574, -6.0929) -> (25.4611, -8.7656)
  line L302 (50.0442, -4.6522) -> (52.1175, -0.9174)
  line L303 (52.1175, -0.9174) -> (56.3885, -0.8456)
  line L304 (52.4291, 14.8875) -> (50.8254, 17.5603)
  line L305 (51.8686, 13.8779) -> (49.6709, 17.5408)
  line L306 (55.5456, 14.9399) -> (52.4291, 14.8875)
  line L307 (58.9315, 9.2967) -> (57.4186, 6.5715)
  line L308 (56.2641, 6.5521) -> (58.3374, 10.2869)
  line L309 (58.3374, 10.2869) -> (56.2641, 6.5521)
  line L310 (49.7953, 10.1432) -> (51.8686, 13.8779)
  line L311 (56.1397, 13.9498) -> (58.3374, 10.2869)
  line L312 (56.1397, 13.9498) -> (58.3374, 10.2869)
  line L313 (58.8979, 11.2964) -> (57.2942, 13.9692)
  line L314 (56.1397, 13.9498) -> (51.8686, 13.8779)
  line L315 (51.8686, 13.8779) -> (56.1397, 13.9498)
  line L316 (59.0223, 3.8987) -> (62.1388, 3.9512)
  line L317 (62.7329, 2.961) -> (58.4619, 2.8892)
  line L318 (62.0144, 11.3489) -> (58.8979, 11.2964)
  line L319 (58.3374, 10.2869) -> (62.5459, 10.3941)
  line L320 (62.048, 9.3491) -> (58.9315, 9.2967)
  line L321 (63.763, 10.3781) -> (65.3667, 7.7054)
  line L322 (64.8062, 6.6958) -> (62.5459, 10.3941)
  line L323 (63.6517, 6.6764) -> (62.048, 9.3491)
  line L324 (62.1388, 3.9512) -> (63.6517, 6.6764)
  line L325 (64.8062, 6.6958) -> (62.7329, 2.961)
  line L326 (65.3667, 7.7054) -> (68.4832, 7.7578)
  line L327 (69.0773, 6.7676) -> (64.8062, 6.6958)
  line L328 (57.4186, 6.5715) -> (59.0223, 3.8987)
  line L329 (57.0584, 17.6651) -> (55.5456, 14.9399)
  line L330 (55.4548, 20.3379) -> (57.0584, 17.6651)
  line L331 (56.0152, 21.3475) -> (58.213, 17.6845)
  line L332 (58.213, 17.6845) -> (56.1397, 13.9498)
  line L333 (51.7442, 21.2756) -> (56.0152, 21.3475)
  line L334 (52.3382, 20.2855) -> (55.4548, 20.3379)
  line L335 (50.8254, 17.5603) -> (52.3382, 20.2855)
  line L336 (57.2942, 13.9692) -> (58.807, 16.6944)
  line L337 (62.484, 17.7564) -> (58.213, 17.6845)
  line L338 (58.807, 16.6944) -> (61.9236, 16.7468)
  line L339 (61.9236, 16.7468) -> (63.5272, 14.0741)
  line L340 (64.6818, 14.0935) -> (62.484, 17.7564)
  line L341 (63.5272, 14.0741) -> (62.0144, 11.3489)
  line L342 (62.5459, 10.3941) -> (64.6818, 14.0935)
  line L343 (63.763, 10.3781) -> (65.2759, 13.1033)
  line L344 (68.3924, 13.1558) -> (65.2759, 13.1033)
  line L345 (68.9528, 14.1653) -> (64.6818, 14.0935)
  line L346 (68.3924, 13.1558) -> (69.996, 10.483)
  line L347 (69.996, 10.483) -> (68.4832, 7.7578)
  line L348 (69.0773, 6.7676) -> (71.1506, 10.5024)
  line L349 (71.1506, 10.5024) -> (68.9528, 14.1653)
  line L350 (43.6998, -8.4588) -> (39.4288, -8.5307)
  line L351 (43.5754, -1.0611) -> (39.3043, -1.133)
  line L352 (43.0149, -2.0707) -> (44.6186, -4.7435)
  line L353 (45.7731, -4.724) -> (43.5754, -1.0611)
  line L354 (43.1057, -7.4687) -> (44.6186, -4.7435)
  line L355 (45.7731, -4.724) -> (43.6998, -8.4588)
  line L356 (45.7731, -4.724) -> (50.0442, -4.6522)
  line L357 (39.9892, -7.5211) -> (43.1057, -7.4687)
  line L358 (38.3856, -4.8483) -> (39.9892, -7.5211)
  line L359 (39.4288, -8.5307) -> (37.231, -4.8677)
  line L360 (38.3856, -4.8483) -> (39.8984, -2.1231)
  line L361 (58.4619, 2.8892) -> (56.3885, -0.8456)
  line L362 (56.2641, 6.5521) -> (58.4619, 2.8892)
  line L363 (45.5242, 10.0713) -> (43.3265, 13.7342)
  line L364 (43.3265, 13.7342) -> (39.0554, 13.6624)
  line L365 (39.0554, 13.6624) -> (36.9821, 9.9276)
  line L366 (43.0149, -2.0707) -> (39.8984, -2.1231)
  line L367 (49.7953, 10.1432) -> (45.5242, 10.0713)
  line L368 (49.7953, 10.1432) -> (45.5242, 10.0713)
  line L369 (45.5242, 10.0713) -> (43.3265, 13.7342)
  line L370 (46.0847, 11.0809) -> (49.2012, 11.1333)
  line L371 (44.481, 13.7537) -> (46.0847, 11.0809)
  line L372 (45.9939, 16.4788) -> (44.481, 13.7537)
  line L373 (43.3265, 13.7342) -> (45.3998, 17.469)
  line L374 (49.2012, 11.1333) -> (50.7141, 13.8585)
  line L375 (49.1104, 16.5313) -> (45.9939, 16.4788)
  line L376 (49.6709, 17.5408) -> (45.3998, 17.469)
  line L377 (50.7141, 13.8585) -> (49.1104, 16.5313)
  line L378 (49.6709, 17.5408) -> (51.8686, 13.8779)
  line L379 (30.3889, 20.9164) -> (32.5866, 17.2534)
  line L380 (32.5866, 17.2534) -> (30.5133, 13.5187)
  line L381 (26.2423, 13.4468) -> (24.0445, 17.1097)
  line L382 (26.8027, 14.4564) -> (25.1991, 17.1292)
  line L383 (29.9192, 14.5088) -> (26.8027, 14.4564)
  line L384 (31.4321, 17.234) -> (29.9192, 14.5088)
  line L385 (29.8284, 19.9068) -> (31.4321, 17.234)
  line L386 (24.0445, 17.1097) -> (26.1178, 20.8445)
  line L387 (26.1178, 20.8445) -> (30.3889, 20.9164)
  line L388 (25.1991, 17.1292) -> (26.7119, 19.8544)
  line L389 (26.7119, 19.8544) -> (29.8284, 19.9068)
  line L390 (24.0445, 17.1097) -> (19.7735, 17.0379)
  line L391 (17.5757, 20.7008) -> (19.7735, 17.0379)
  line L392 (23.9201, 24.5074) -> (19.649, 24.4356)
  line L393 (18.7303, 20.7202) -> (20.3339, 18.0475)
  line L394 (20.3339, 18.0475) -> (23.4504, 18.0999)
  line L395 (23.4504, 18.0999) -> (24.9633, 20.8251)
  line L396 (24.9633, 20.8251) -> (23.3596, 23.4979)
  line L397 (26.1178, 20.8445) -> (23.9201, 24.5074)
  line L398 (23.3596, 23.4979) -> (20.2431, 23.4454)
  line L399 (20.2431, 23.4454) -> (18.7303, 20.7202)
  line L400 (19.649, 24.4356) -> (17.5757, 20.7008)
  line L401 (32.4622, 24.6511) -> (30.3889, 20.9164)
  line L402 (30.2644, 28.314) -> (32.4622, 24.6511)
  line L403 (30.3889, 20.9164) -> (26.1178, 20.8445)
  line L404 (29.7948, 21.9065) -> (26.6783, 21.8541)
  line L405 (26.6783, 21.8541) -> (25.0746, 24.5269)
  line L406 (23.9201, 24.5074) -> (25.9934, 28.2422)
  line L407 (25.0746, 24.5269) -> (26.5875, 27.252)
  line L408 (25.9934, 28.2422) -> (30.2644, 28.314)
  line L409 (26.5875, 27.252) -> (29.704, 27.3045)
  line L410 (29.704, 27.3045) -> (31.3077, 24.6317)
  line L411 (31.3077, 24.6317) -> (29.7948, 21.9065)
  line L412 (13.3047, 20.629) -> (11.1069, 24.2919)
  line L413 (17.5757, 20.7008) -> (13.3047, 20.629)
  line L414 (11.1069, 24.2919) -> (13.1802, 28.0266)
  line L415 (12.2615, 24.3113) -> (13.7743, 27.0365)
  line L416 (13.7743, 27.0365) -> (16.8908, 27.0889)
  line L417 (13.1802, 28.0266) -> (17.4513, 28.0985)
  line L418 (17.4513, 28.0985) -> (19.649, 24.4356)
  line L419 (16.8908, 27.0889) -> (18.4945, 24.4162)
  line L420 (18.4945, 24.4162) -> (16.9816, 21.691)
  line L421 (16.9816, 21.691) -> (13.8651, 21.6385)
  line L422 (13.8651, 21.6385) -> (12.2615, 24.3113)
  line L423 (23.9201, 24.5074) -> (25.9934, 28.2422)
  line L424 (23.7956, 31.9051) -> (25.9934, 28.2422)
  line L425 (19.649, 24.4356) -> (23.9201, 24.5074)
  line L426 (20.2095, 25.4452) -> (23.326, 25.4976)
  line L427 (18.6058, 28.1179) -> (20.2095, 25.4452)
  line L428 (19.5246, 31.8333) -> (17.4513, 28.0985)
  line L429 (20.1187, 30.8431) -> (18.6058, 28.1179)
  line L430 (23.7956, 31.9051) -> (19.5246, 31.8333)
  line L431 (23.2352, 30.8955) -> (20.1187, 30.8431)
  line L432 (24.8389, 28.2228) -> (23.2352, 30.8955)
  line L433 (23.326, 25.4976) -> (24.8389, 28.2228)
  line L434 (4.7626, 20.4853) -> (6.9603, 16.8224)
  line L435 (4.7626, 20.4853) -> (0.4915, 20.4134)
  line L436 (-1.5818, 16.6787) -> (0.616, 13.0157)
  line L437 (-5.8528, 16.6068) -> (-1.5818, 16.6787)
  line L438 (-1.7062, 24.0763) -> (0.4915, 20.4134)
  line L439 (-7.9261, 12.872) -> (-5.8528, 16.6068)
  line L440 (-12.1972, 12.8002) -> (-7.9261, 12.872)
  line L441 (-12.0195, 13.8033) -> (-13.7923, 16.7581)
  line L442 (-14.395, 16.4631) -> (-12.1972, 12.8002)
  line L443 (-12.3216, 20.1979) -> (-14.395, 16.4631)
  line L444 (-13.7923, 16.7581) -> (-12.272, 19.4967)
  line L445 (-1.8307, 31.474) -> (-6.1017, 31.4022)
  line L446 (0.3671, 27.8111) -> (-1.8307, 31.474)
  line L447 (-1.7062, 24.0763) -> (0.3671, 27.8111)
  line L448 (13.1802, 28.0266) -> (10.9825, 31.6896)
  line L449 (7.3963, 25.2296) -> (5.7927, 27.9024)
  line L450 (10.5128, 25.282) -> (7.3963, 25.2296)
  line L451 (5.7927, 27.9024) -> (7.3055, 30.6276)
  line L452 (12.0257, 28.0072) -> (10.5128, 25.282)
  line L453 (10.422, 30.68) -> (12.0257, 28.0072)
  line L454 (7.3055, 30.6276) -> (10.422, 30.68)
  line L455 (4.6381, 27.883) -> (6.8359, 24.22)
  line L456 (6.7114, 31.6177) -> (10.9825, 31.6896)
  line L457 (13.1802, 28.0266) -> (11.1069, 24.2919)
  line L458 (4.6381, 27.883) -> (6.7114, 31.6177)
  line L459 (0.3671, 27.8111) -> (-1.7062, 24.0763)
  line L460 (5.6813, 24.2006) -> (4.1685, 21.4754)
  line L461 (4.0777, 26.8734) -> (5.6813, 24.2006)
  line L462 (4.1685, 21.4754) -> (1.052, 21.423)
  line L463 (6.8359, 24.22) -> (4.6381, 27.883)
  line L464 (0.9612, 26.821) -> (4.0777, 26.8734)
  line L465 (-0.5517, 24.0958) -> (0.9612, 26.821)
  line L466 (1.052, 21.423) -> (-0.5517, 24.0958)
  line L467 (-1.7062, 24.0763) -> (0.4915, 20.4134)
  line L468 (0.4915, 20.4134) -> (4.7626, 20.4853)
  line L469 (4.6381, 27.883) -> (0.3671, 27.8111)
  line L470 (4.5137, 35.2806) -> (6.7114, 31.6177)
  line L471 (4.5137, 35.2806) -> (0.2426, 35.2088)
  line L472 (-1.8307, 31.474) -> (0.2426, 35.2088)
  line L473 (5.5569, 31.5983) -> (3.9532, 34.2711)
  line L474 (6.7114, 31.6177) -> (4.6381, 27.883)
  line L475 (0.9275, 28.8207) -> (4.044, 28.8731)
  line L476 (0.3671, 27.8111) -> (-1.8307, 31.474)
  line L477 (-0.6761, 31.4934) -> (0.9275, 28.8207)
  line L478 (3.9532, 34.2711) -> (0.8367, 34.2186)
  line L479 (19.5246, 31.8333) -> (17.3268, 35.4962)
  line L480 (18.37, 31.8138) -> (16.7664, 34.4866)
  line L481 (16.8572, 29.0886) -> (18.37, 31.8138)
  line L482 (17.4513, 28.0985) -> (19.5246, 31.8333)
  line L483 (13.7407, 29.0362) -> (16.8572, 29.0886)
  line L484 (10.9825, 31.6896) -> (13.1802, 28.0266)
  line L485 (12.137, 31.709) -> (13.7407, 29.0362)
  line L486 (13.6499, 34.4342) -> (12.137, 31.709)
  line L487 (13.0558, 35.4243) -> (10.9825, 31.6896)
  line L488 (16.7664, 34.4866) -> (13.6499, 34.4342)
  line L489 (17.3268, 35.4962) -> (13.0558, 35.4243)
  line L490 (32.3377, 32.0488) -> (30.2644, 28.314)
  line L491 (25.8689, 35.6399) -> (30.14, 35.7117)
  line L492 (25.8689, 35.6399) -> (23.7956, 31.9051)
  line L493 (26.5538, 29.2518) -> (29.6704, 29.3042)
  line L494 (24.9502, 31.9245) -> (26.5538, 29.2518)
  line L495 (23.7956, 31.9051) -> (25.9934, 28.2422)
  line L496 (26.463, 34.6497) -> (24.9502, 31.9245)
  line L497 (29.5795, 34.7022) -> (26.463, 34.6497)
  line L498 (32.3377, 32.0488) -> (30.14, 35.7117)
  line L499 (31.1832, 32.0294) -> (29.5795, 34.7022)
  line L500 (29.6704, 29.3042) -> (31.1832, 32.0294)
  line L501 (42.9532, 35.9273) -> (38.6821, 35.8554)
  line L502 (39.2762, 34.8653) -> (42.3927, 34.9177)
  line L503 (37.7633, 32.1401) -> (39.2762, 34.8653)
  line L504 (38.6821, 35.8554) -> (36.6088, 32.1207)
  line L505 (45.1509, 32.2644) -> (42.9532, 35.9273)
  line L506 (42.3927, 34.9177) -> (43.9964, 32.2449)
  line L507 (43.0776, 28.5296) -> (45.1509, 32.2644)
  line L508 (43.9964, 32.2449) -> (42.4835, 29.5197)
  line L509 (42.4835, 29.5197) -> (39.367, 29.4673)
  line L510 (39.367, 29.4673) -> (37.7633, 32.1401)
  line L511 (36.6088, 32.1207) -> (38.8065, 28.4577)
  line L512 (49.5464, 24.9385) -> (51.6197, 28.6733)
  line L513 (50.4652, 28.6539) -> (48.9523, 25.9287)
  line L514 (48.8615, 31.3266) -> (50.4652, 28.6539)
  line L515 (51.6197, 28.6733) -> (49.4226, 32.2644)
  line L516 (45.2754, 24.8667) -> (49.5464, 24.9385)
  line L517 (48.9523, 25.9287) -> (45.8358, 25.8762)
  line L518 (45.8358, 25.8762) -> (44.2321, 28.549)
  line L519 (44.2321, 28.549) -> (45.745, 31.2742)
  line L520 (45.1509, 32.2644) -> (43.0776, 28.5296)
  line L521 (45.745, 31.2742) -> (48.8615, 31.3266)
  line L522 (49.4226, 32.2644) -> (45.1509, 32.2644)
  line L523 (56.934, 25.0628) -> (55.4211, 22.3376)
  line L524 (58.0885, 25.0822) -> (56.0152, 21.3475)
  line L525 (55.3303, 27.7356) -> (56.934, 25.0628)
  line L526 (55.8908, 28.7451) -> (58.0885, 25.0822)
  line L527 (52.2138, 27.6831) -> (55.3303, 27.7356)
  line L528 (50.7009, 24.9579) -> (52.2138, 27.6831)
  line L529 (49.5464, 24.9385) -> (51.6197, 28.6733)
  line L530 (51.6197, 28.6733) -> (55.8908, 28.7451)
  line L531 (52.3046, 22.2852) -> (50.7009, 24.9579)
  line L532 (55.4211, 22.3376) -> (52.3046, 22.2852)
  line L533 (56.0152, 21.3475) -> (51.7442, 21.2756)
  line L534 (64.4329, 28.8888) -> (62.2351, 32.5518)
  line L535 (64.4329, 28.8888) -> (62.3596, 25.1541)
  line L536 (62.2351, 32.5518) -> (57.9641, 32.4799)
  line L537 (63.2783, 28.8694) -> (61.6747, 31.5422)
  line L538 (61.6747, 31.5422) -> (58.5582, 31.4898)
  line L539 (57.9641, 32.4799) -> (55.8908, 28.7451)
  line L540 (58.5582, 31.4898) -> (57.0453, 28.7646)
  line L541 (57.0453, 28.7646) -> (58.649, 26.0918)
  line L542 (58.0885, 25.0822) -> (62.3596, 25.1541)
  line L543 (58.649, 26.0918) -> (61.7655, 26.1442)
  line L544 (61.7655, 26.1442) -> (63.2783, 28.8694)
  line L545 (62.3596, 25.1541) -> (58.0885, 25.0822)
  line L546 (63.4028, 21.4717) -> (61.7991, 24.1445)
  line L547 (64.5573, 21.4912) -> (62.3596, 25.1541)
  line L548 (61.8899, 18.7465) -> (63.4028, 21.4717)
  line L549 (62.484, 17.7564) -> (64.5573, 21.4912)
  line L550 (61.7991, 24.1445) -> (58.6826, 24.0921)
  line L551 (58.7734, 18.6941) -> (61.8899, 18.7465)
  line L552 (58.213, 17.6845) -> (62.484, 17.7564)
  line L553 (57.1697, 21.3669) -> (58.7734, 18.6941)
  line L554 (58.6826, 24.0921) -> (57.1697, 21.3669)
  line L555 (58.0885, 25.0822) -> (56.0152, 21.3475)
  line L556 (63.8874, 2.9805) -> (65.4911, 0.3077)
  line L557 (62.7329, 2.961) -> (64.9307, -0.7019)
  line L558 (69.2017, -0.63) -> (64.9307, -0.7019)
  line L559 (68.6076, 0.3601) -> (65.4911, 0.3077)
  line L560 (63.8874, 2.9805) -> (65.4003, 5.7056)
  line L561 (65.4003, 5.7056) -> (68.5168, 5.7581)
  line L562 (70.1205, 3.0853) -> (68.5168, 5.7581)
  line L563 (68.6076, 0.3601) -> (70.1205, 3.0853)
  line L564 (71.275, 3.1047) -> (69.2017, -0.63)
  line L565 (69.0773, 6.7676) -> (71.275, 3.1047)
  line L566 (64.8062, 6.6958) -> (62.7329, 2.961)
  line L567 (63.6386, 17.7758) -> (65.2422, 15.103)
  line L568 (62.484, 17.7564) -> (64.6818, 14.0935)
  line L569 (68.3587, 15.1555) -> (65.2422, 15.103)
  line L570 (63.6386, 17.7758) -> (65.1514, 20.501)
  line L571 (65.1514, 20.501) -> (68.2679, 20.5534)
  line L572 (69.8716, 17.8807) -> (68.2679, 20.5534)
  line L573 (68.3587, 15.1555) -> (69.8716, 17.8807)
  line L574 (71.0261, 17.9001) -> (68.9528, 14.1653)
  line L575 (68.8284, 21.563) -> (71.0261, 17.9001)
  line L576 (68.8284, 21.563) -> (64.5573, 21.4912)
  line L577 (64.5573, 21.4912) -> (62.484, 17.7564)
  line L578 (64.4329, 28.8888) -> (62.3596, 25.1541)
  line L579 (68.7039, 28.9607) -> (64.4329, 28.8888)
  line L580 (65.1178, 22.5007) -> (68.2343, 22.5532)
  line L581 (63.5141, 25.1735) -> (65.1178, 22.5007)
  line L582 (64.5573, 21.4912) -> (62.3596, 25.1541)
  line L583 (63.5141, 25.1735) -> (65.027, 27.8987)
  line L584 (68.1435, 27.9511) -> (65.027, 27.8987)
  line L585 (70.9017, 25.2978) -> (68.7039, 28.9607)
  line L586 (68.1435, 27.9511) -> (69.7471, 25.2784)
  line L587 (69.7471, 25.2784) -> (68.2343, 22.5532)
  line L588 (68.8284, 21.563) -> (70.9017, 25.2978)
  line L589 (64.4329, 28.8888) -> (62.2351, 32.5518)
  line L590 (64.3084, 36.2865) -> (62.2351, 32.5518)
  line L591 (68.5795, 36.3584) -> (64.3084, 36.2865)
  line L592 (68.1098, 29.9508) -> (64.9933, 29.8984)
  line L593 (63.3897, 32.5712) -> (64.9933, 29.8984)
  line L594 (63.3897, 32.5712) -> (64.9025, 35.2964)
  line L595 (64.9025, 35.2964) -> (68.019, 35.3488)
  line L596 (68.5795, 36.3584) -> (70.7772, 32.6955)
  line L597 (69.6227, 32.676) -> (68.019, 35.3488)
  line L598 (68.1098, 29.9508) -> (69.6227, 32.676)
  line L599 (70.7772, 32.6955) -> (68.7039, 28.9607)
  line L600 (51.4953, 36.071) -> (49.422, 32.3362)
  line L601 (51.4953, 36.071) -> (55.7663, 36.1428)
  line L602 (52.0894, 35.0808) -> (50.5765, 32.3556)
  line L603 (50.5765, 32.3556) -> (52.1802, 29.6829)
  line L604 (49.422, 32.3362) -> (51.6197, 28.6733)
  line L605 (52.1802, 29.6829) -> (55.2967, 29.7353)
  line L606 (55.2967, 29.7353) -> (56.8095, 32.4605)
  line L607 (55.8908, 28.7451) -> (57.9641, 32.4799)
  line L608 (57.9641, 32.4799) -> (55.7663, 36.1428)
  line L609 (56.8095, 32.4605) -> (55.2059, 35.1333)
  line L610 (55.2059, 35.1333) -> (52.0894, 35.0808)
  line L611 (-1.084, -12.9121) -> (1.1137, -16.575)
  line L612 (1.1137, -16.575) -> (5.3848, -16.5031)
  line L613 (5.3848, -16.5031) -> (7.4581, -12.7684)
  line L614 (7.4581, -12.7684) -> (5.2604, -9.1055)
  line L615 (5.2604, -9.1055) -> (0.9893, -9.1773)
  line L616 (0.0705, -12.8926) -> (1.6742, -15.5654)
  line L617 (1.6742, -15.5654) -> (4.7907, -15.513)
  line L618 (4.7907, -15.513) -> (6.3036, -12.7878)
  line L619 (6.3036, -12.7878) -> (4.6999, -10.115)
  line L620 (4.6999, -10.115) -> (1.5834, -10.1675)
  line L621 (1.5834, -10.1675) -> (0.0705, -12.8926)
  line L622 (11.7292, -12.6965) -> (7.4581, -12.7684)
  line L623 (11.7292, -12.6965) -> (13.8025, -8.9618)
  line L624 (11.6047, -5.2988) -> (13.8025, -8.9618)
  line L625 (11.6047, -5.2988) -> (7.3337, -5.3707)
  line L626 (11.0443, -6.3084) -> (7.9277, -6.3608)
  line L627 (12.6479, -8.9812) -> (11.0443, -6.3084)
  line L628 (11.1351, -11.7064) -> (12.6479, -8.9812)
  line L629 (8.0186, -11.7588) -> (11.1351, -11.7064)
  line L630 (6.4149, -9.086) -> (8.0186, -11.7588)
  line L631 (7.9277, -6.3608) -> (6.4149, -9.086)
  line L632 (5.2604, -9.1055) -> (7.4581, -12.7684)
  line L633 (13.9269, -16.3594) -> (11.8536, -20.0942)
  line L634 (7.5825, -20.1661) -> (11.8536, -20.0942)
  line L635 (11.7292, -12.6965) -> (13.9269, -16.3594)
  line L636 (12.7724, -16.3789) -> (11.2595, -19.1041)
  line L637 (11.2595, -19.1041) -> (8.143, -19.1565)
  line L638 (8.143, -19.1565) -> (6.5393, -16.4837)
  line L639 (7.5825, -20.1661) -> (5.3848, -16.5031)
  line L640 (6.5393, -16.4837) -> (8.0522, -13.7585)
  line L641 (7.4581, -12.7684) -> (11.7292, -12.6965)
  line L642 (8.0522, -13.7585) -> (11.1687, -13.7061)
  line L643 (11.7292, -12.6965) -> (13.9269, -16.3594)
  line L644 (11.1687, -13.7061) -> (12.7724, -16.3789)
  line L645 (18.0735, -8.8899) -> (13.8025, -8.9618)
  line L646 (11.7292, -12.6965) -> (13.8025, -8.9618)
  line L647 (17.5131, -9.8995) -> (14.3965, -9.9519)
  line L648 (20.2713, -12.5528) -> (18.0735, -8.8899)
  line L649 (19.1167, -12.5722) -> (17.5131, -9.8995)
  line L650 (17.6039, -15.2974) -> (19.1167, -12.5722)
  line L651 (20.2713, -12.5528) -> (18.198, -16.2876)
  line L652 (14.4874, -15.3499) -> (17.6039, -15.2974)
  line L653 (13.9269, -16.3594) -> (18.198, -16.2876)
  line L654 (12.8837, -12.6771) -> (14.4874, -15.3499)
  line L655 (14.3965, -9.9519) -> (12.8837, -12.6771)
  line L656 (18.3224, -23.6853) -> (20.3957, -19.9505)
  line L657 (18.198, -16.2876) -> (20.3957, -19.9505)
  line L658 (17.7283, -22.6951) -> (19.2412, -19.9699)
  line L659 (14.0514, -23.7571) -> (18.3224, -23.6853)
  line L660 (14.6118, -22.7476) -> (17.7283, -22.6951)
  line L661 (13.0081, -20.0748) -> (14.6118, -22.7476)
  line L662 (14.0514, -23.7571) -> (11.8536, -20.0942)
  line L663 (14.521, -17.3496) -> (13.0081, -20.0748)
  line L664 (18.198, -16.2876) -> (13.9269, -16.3594)
  line L665 (17.6375, -17.2972) -> (14.521, -17.3496)
  line L666 (19.2412, -19.9699) -> (17.6375, -17.2972)
  line L667 (5.3848, -16.5031) -> (1.1137, -16.575)
  line L668 (4.8243, -17.5127) -> (1.7078, -17.5651)
  line L669 (6.428, -20.1855) -> (4.8243, -17.5127)
  line L670 (4.9152, -22.9107) -> (6.428, -20.1855)
  line L671 (7.5825, -20.1661) -> (5.5092, -23.9008)
  line L672 (1.7986, -22.9631) -> (4.9152, -22.9107)
  line L673 (1.2382, -23.9727) -> (5.5092, -23.9008)
  line L674 (-0.9596, -20.3098) -> (1.2382, -23.9727)
  line L675 (0.195, -20.2903) -> (1.7986, -22.9631)
  line L676 (1.7078, -17.5651) -> (0.195, -20.2903)
  line L677 (1.1137, -16.575) -> (-0.9596, -20.3098)
  line L678 (5.5092, -23.9008) -> (7.707, -27.5637)
  line L679 (11.978, -27.4919) -> (7.707, -27.5637)
  line L680 (6.6638, -23.8814) -> (8.2674, -26.5542)
  line L681 (7.5825, -20.1661) -> (5.5092, -23.9008)
  line L682 (8.1766, -21.1562) -> (6.6638, -23.8814)
  line L683 (11.2932, -21.1038) -> (8.1766, -21.1562)
  line L684 (12.8968, -23.7765) -> (11.2932, -21.1038)
  line L685 (14.0514, -23.7571) -> (11.8536, -20.0942)
  line L686 (11.978, -27.4919) -> (14.0514, -23.7571)